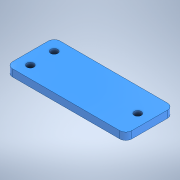
# Autodesk Inventor part: EboxTslotMount
Saved by Autodesk Inventor 2022 (Build 260153000, 153)
## iProperties
Created: 2022-02-24
Part Number: EboxTslotMount
Material: Generic
Document SubType Name: Modeling
Designer: Jorian Brusind
Density: 1 g/cm^3
Appearance: Cyan
Author: Jorian Brusind
Autodesk Inventor part; units mm, degrees
ref_plane "YZ Plane" through (0, 0, 0) normal (1, 0, 0) x (0, 1, 0)
ref_plane "XZ Plane" through (0, 0, 0) normal (0, 1, 0) x (-1, 0, 0)
ref_plane "XY Plane" through (0, 0, 0) normal (0, 0, 1) x (1, 0, 0)
sketch "Sketch1" plane through (0, 0, 0) normal (0, 1, 0) x (-1, 0, 0)
  line L0 (0, 0) -> (100, 0)
  line L1 (100, 0) -> (100, -40)
  line L2 (100, -40) -> (0, -40)
  line L3 (0, -40) -> (0, 0)
  circle A0 centre (10, -20) radius 3
  circle A1 centre (90, -10) radius 3
  circle A2 centre (90, -30) radius 3
  dimension "d0" = 100
  dimension "d1" = 40
  dimension "d2" = 6
  dimension "d3" = 10
  dimension "d4" = 20
  dimension "d5" = 6
  dimension "d6" = 10
  dimension "d7" = 6
  dimension "d8" = 20
  dimension "d9" = 10
  dimension "d10" = 10
  constraints: 8 end point, 3 centre point, 2 parallel, 1 horizontal, 1 perpendicular
  measures "d0" distance of L1.end L2.end
  measures "d1" distance of L0.end L1.end
  measures "d2" diameter of A0
  measures "d3" distance from line of L3 A0.centre
  measures "d4" distance from line of L0 A0.centre
  measures "d5" diameter of A1
  measures "d6" distance from line of L0 A1.centre
  measures "d7" diameter of A2
  measures "d8" distance of A2.centre A1.centre
  measures "d9" distance from line of L2 A2.centre
  measures "d10" distance from line of L1 A2.centre
extrude "Extrusion1" add sketch "Sketch1" along normal blind 6
fillet "Fillet1" radius 5 4 edges at (0, 3, 0) (0, 3, -40) (-100, 3, 0) (-100, 3, -40)
body "Solid1"
